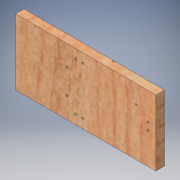
# Autodesk Inventor part: Sun_BaseStaple
Saved by Autodesk Inventor 2016 (Build 200138000, 138)
## iProperties
Created: 2017-11-14
Part Number: Sun_BaseStaple
Material: Wood (Birch)
Document SubType Name: Modeling
Designer: sun01147
Density: 0.55 g/cm^3
Appearance: Birch - Natural Polished
Author: sun01147
Autodesk Inventor part; units mm, degrees
ref_plane "YZ Plane" through (0, 0, 0) normal (1, 0, 0) x (0, 1, 0)
ref_plane "XY Plane" through (0, 0, 0) normal (0, 0, 1) x (1, 0, 0)
sketch "Sketch1" plane through (0, 0, 0) normal (0, 0, 1) x (1, 0, 0)
  line L0 (0, 46.2534) -> (98.425, 46.2534)
  line L1 (98.425, 46.2534) -> (98.425, 0)
  line L2 (98.425, 0) -> (0, 0)
  line L3 (0, 0) -> (0, 46.2534)
  point P0 (0, 0)
  dimension "d0" = 98.425
  dimension "d1" = 46.2534
  constraints: 8 end point, 2 coincident, 2 parallel, 1 horizontal, 1 perpendicular
  measures "d0" distance of L0.start L0.end
  measures "d1" distance of L0.end L1.end
extrude "Extrusion1" add sketch "Sketch1" against normal blind 5.969
sketch "Sketch2" plane through (0, 0, 0) normal (0, 0, 1) x (1, 0, 0)
  line L0 (0, 0) -> (0, 46.2534) projected
  line L1 (98.425, 0) -> (0, 0) projected
  line L2 (98.425, 46.2534) -> (98.425, 0) projected
  line L3 (0, 46.2534) -> (98.425, 46.2534) projected
  point P0 (42.164, 39.9034)
  point P1 (47.117, 39.9034)
  point P2 (36.0426, 31.6992)
  point P3 (36.0426, 14.5542)
  point P4 (42.164, 6.35)
  point P5 (47.117, 6.35)
  point P6 (92.964, 26.8478)
  point P7 (92.964, 21.8948)
  dimension "d22" = 42.164
  dimension "d23" = 36.0426
  dimension "d24" = 14.5542
  dimension "d25" = 36.0426
  dimension "d26" = 47.117
  dimension "d27" = 42.164
  dimension "d29" = 5.461
  dimension "d32" = 19.4056
  dimension "d33" = 6.35
  dimension "d34" = 6.35
  dimension "d35" = 14.5542
  dimension "d36" = 6.35
  dimension "d37" = 6.35
  dimension "d38" = 4.953
  dimension "d39" = 17.145
  dimension "d40" = 5.461
  dimension "d41" = 4.953
  measures "d22" distance from line of L0 point (42.164, 39.903)
  measures "d23" distance from line of L0 point (36.043, 31.699)
  measures "d24" distance from line of L1 point (36.043, 14.554)
  measures "d25" distance from line of L0 point (36.043, 14.554)
  measures "d26" distance from line of L0 point (47.117, 6.35)
  measures "d27" distance from line of L0 point (42.164, 6.35)
  measures "d29" distance from line of L2 point (92.964, 26.848)
  measures "d32" distance from line of L3 point (92.964, 26.848)
  measures "d33" distance from line of L3 point (47.117, 39.903)
  measures "d34" distance from line of L3 point (42.164, 39.903)
  measures "d35" distance from line of L3 point (36.043, 31.699)
  measures "d36" distance from line of L1 point (42.164, 6.35)
  measures "d37" distance from line of L1 point (47.117, 6.35)
  measures "d38" distance of point (47.117, 39.903) point (42.164, 39.903)
  measures "d39" distance of point (36.043, 14.554) point (36.043, 31.699)
  measures "d40" distance from line of L2 point (92.964, 21.895)
  measures "d41" distance of point (92.964, 26.848) point (92.964, 21.895)
hole "Hole1" at (42.164, 39.9034, 0) at (47.117, 39.9034, 0) at (36.0426, 31.6992, 0) at (36.0426, 14.5542, 0) at (42.164, 6.35, 0) at (47.117, 6.35, 0) at (92.964, 26.8478, 0) at (92.964, 21.8948, 0) direction (0, 0, -1) diameter 1.397 end through all
body "Solid1"
